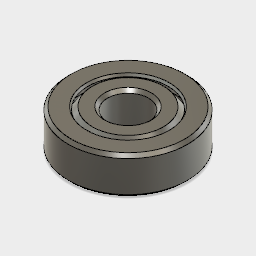
f1-bearing-625 (Autodesk Fusion 360 design; units mm, degrees)
Autodesk Fusion 360 part; units mm, degrees
sketch "Skizze1" plane through (0, 0, 0) normal (1, 0, 0) x (0, 0, -1)
  line L0 (-2.75, -0.5) -> (-2.75, -5.5)
  line L1 (-8, -5.5) -> (-8, -0.5)
  line L2 (-5.1411, -0.5) -> (-6.3214, -2.25)
  line L3 (-6.3214, -2.25) -> (-6.3214, -3.75)
  line L4 (-6.3214, -3.75) -> (-5.1411, -5.5)
  line L5 (-6.0214, -3.75) -> (-6.0214, -2.25)
  line L6 (-6.0214, -2.25) -> (-4.75, -0.5)
  line L7 (-2.75, -5.5) -> (-4.75, -5.5)
  line L8 (-5.1411, -5.5) -> (-8, -5.5)
  line L9 (-8, -0.5) -> (-5.1411, -0.5)
  line L10 (-4.75, -0.5) -> (-2.75, -0.5)
  line L11 (-6.0214, -3.75) -> (-4.75, -5.5)
  line L12 (0, 0) -> (0, -7.2054)
  dimension "d2" = 2.75
  dimension "d3" = 5
  dimension "d4" = 8
  dimension "d5" = 1.5
  dimension "d6" = 1.5
  dimension "d7" = 1.75
  dimension "d8" = 1.75
  dimension "d9" = 56
  dimension "d10" = 56
  dimension "d11" = 0.3
  dimension "d12" = 54
  dimension "d14" = 54
  dimension "d15" = 1.5714
  dimension "d20" = 2
  measures "d2" distance of L12.start L0
  measures "d3" distance of L1.end L1.start
  measures "d4" distance of L12.start L1
  measures "d5" distance of L2.end L3.end
  measures "d6" distance of L5.start L5.end
  measures "d7" distance of L3.end L8
  measures "d8" distance of L5.start L7
  measures "d9" angle of L2 L9
  measures "d10" angle of L4 L8
  measures "d11" distance of L3 L5
  measures "d12" angle of L6 L10
  measures "d14" angle of L8 L11
  measures "d15" distance of L3 L7.end
  measures "d20" distance of L0.end L7.end
revolve "Drehen1" add sketch "Skizze1" angle 360 about axis through (0, 0, 0) along (0, -1, 0) makes body 1 at (0.3988, -3.8333, 7.9901) makes body 2 at (0.2738, -2.1667, 2.7363)
chamfer "Fase1" distance 0.4 angle 45 6 edges at (-2.5639, -0.5, 0.9944) (-2.5639, -5.5, 0.9944) (-4.7932, -0.5, 1.8591) (-7.4586, -0.5, 2.8929) (-7.4586, -5.5, 2.8929) (-4.7932, -5.5, 1.8591) on bodies 1 2
equation "d2 = ( 5.5 / 2 ) * 1 mm"
equation "d4 = ( 16 / 2 ) * 1 mm"
equation "d6 = d5"
equation "d7 = ( d3 - d5 ) / 2"
equation "d8 = d7"
equation "d10 = d9"
equation "d14 = d12"
